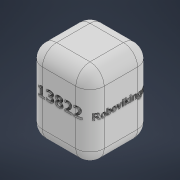
# Autodesk Inventor part: Robovikings Basic Capstone
Saved by Autodesk Inventor 2022 (Build 260153000, 153)
## iProperties
Created: 2022-01-25
Part Number: Robovikings Basic Capstone
Material: Generic
Document SubType Name: Modeling
Designer: izack
Density: 1 g/cm^3
Appearance: Default
Author: izack
Autodesk Inventor part; units mm, degrees
(part 1 of 2)
ref_plane "YZ Plane" through (0, 0, 0) normal (1, 0, 0) x (0, 1, 0)
ref_plane "XZ Plane" through (0, 0, 0) normal (0, 1, 0) x (-1, 0, 0)
ref_plane "XY Plane" through (0, 0, 0) normal (0, 0, 1) x (1, 0, 0)
sketch "Sketch1" plane through (0, 0, 0) normal (0, 1, 0) x (-1, 0, 0)
  line L0 (0, 0) -> (76.2, 0)
  line L1 (76.2, 0) -> (76.2, -76.2)
  line L2 (76.2, -76.2) -> (0, -76.2)
  line L3 (0, -76.2) -> (0, 0)
  dimension "d0" = 76.2
  dimension "d1" = 76.2
  constraints: 8 end point, 2 parallel, 1 horizontal, 1 perpendicular
  measures "d0" distance of L1.end L2.end
  measures "d1" distance of L0.end L1.end
extrude "Extrusion1" add sketch "Sketch1" along normal blind 101.6
shell "Shell1" thickness 12.7 removed faces 1 at (-25.4, 0, -25.4)
fillet "Fillet1" radius 17.4625 20 edges at (-38.1, 88.9, -63.5) (-63.5, 88.9, -38.1) (-63.5, 44.45, -63.5) (-63.5, 44.45, -12.7) (-12.7, 88.9, -38.1) (-38.1, 88.9, -12.7) (-12.7, 44.45, -63.5) (-12.7, 44.45, -12.7) (-38.1, 0, -76.2) (-76.2, 0, -38.1) (-38.1, 0, 0) (0, 0, -38.1) (-76.2, 50.8, -76.2) (-38.1, 101.6, -76.2) (-76.2, 101.6, -38.1) (0, 50.8, -76.2) (-76.2, 50.8, 0) (0, 50.8, 0) (-38.1, 101.6, 0) (0, 101.6, -38.1)
sketch "Sketch2" plane through (-76.2, 17.4625, -17.4625) normal (-1, 0, 0) x (0, 0, 1)
  line L0 (-41.275, 66.675) -> (-41.275, 0) projected
  line L1 (0, 0) -> (0, 66.675) projected
  line L2 (-41.275, 0) -> (-41.275, 66.675) projected
  line L3 (-41.275, 33.3375) -> (0, 33.3375)
  line L4 (-45.0845, 33.3375) -> (-47.4125, 33.3375)
  line L5 (-47.4125, 33.3375) -> (-49.5305, 36.1348)
  line L6 (-49.5305, 36.1348) -> (-50.2221, 36.1348)
  line L7 (-50.2221, 36.1348) -> (-50.2221, 33.3375)
  line L8 (-50.2221, 33.3375) -> (-52.124, 33.3375)
  line L9 (-52.124, 33.3375) -> (-52.124, 40.9575)
  line L10 (-52.124, 40.9575) -> (-49.0612, 40.9575)
  spline S0 degree 2 poles (-49.0612, 40.9575) (-48.4252, 40.9575) (-47.4866, 40.7969) (-47.0852, 40.5499) knots 0 0 0 1 2 2 2
  spline S1 degree 2 poles (-47.0852, 40.5499) (-46.6776, 40.2906) (-46.196, 39.4817) (-46.196, 38.8642) knots 0 0 0 1 2 2 2
  spline S2 degree 2 poles (-46.196, 38.8642) (-46.196, 37.9935) (-46.9864, 36.9005) (-47.6471, 36.5794) knots 0 0 0 1 2 2 2
  line L11 (-47.6471, 36.5794) -> (-45.0845, 33.3375)
  spline S3 degree 2 poles (-48.1597, 38.6233) (-48.1597, 38.9136) (-48.382, 39.3273) (-48.6351, 39.4384) knots 0 0 0 1 2 2 2
  spline S4 degree 2 poles (-48.6351, 39.4384) (-48.8142, 39.5125) (-49.2526, 39.5558) (-49.5799, 39.5558) knots 0 0 0 1 2 2 2
  line L12 (-49.5799, 39.5558) -> (-50.2221, 39.5558)
  line L13 (-50.2221, 39.5558) -> (-50.2221, 37.5057)
  line L14 (-50.2221, 37.5057) -> (-49.6725, 37.5057)
  spline S5 degree 2 poles (-49.6725, 37.5057) (-49.2773, 37.5057) (-48.7154, 37.6045) (-48.524, 37.7588) knots 0 0 0 1 2 2 2
  spline S6 degree 2 poles (-48.524, 37.7588) (-48.3387, 37.907) (-48.1597, 38.3022) (-48.1597, 38.6233) knots 0 0 0 1 2 2 2
  spline S7 degree 2 poles (-39.107, 36.2089) (-39.107, 34.7886) (-40.657, 33.1584) (-42.0711, 33.1584) knots 0 0 0 1 2 2 2
  spline S8 degree 2 poles (-42.0711, 33.1584) (-43.479, 33.1584) (-45.0413, 34.7886) (-45.0413, 36.2089) knots 0 0 0 1 2 2 2
  spline S9 degree 2 poles (-45.0413, 36.2089) (-45.0413, 37.6415) (-43.479, 39.2655) (-42.0711, 39.2655) knots 0 0 0 1 2 2 2
  spline S10 degree 2 poles (-42.0711, 39.2655) (-40.6632, 39.2655) (-39.107, 37.6353) (-39.107, 36.2089) knots 0 0 0 1 2 2 2
  spline S11 degree 2 poles (-40.941, 36.1965) (-40.941, 36.7091) (-41.1078, 37.3945) (-41.256, 37.5983) knots 0 0 0 1 2 2 2
  spline S12 degree 2 poles (-41.256, 37.5983) (-41.4165, 37.8144) (-41.8179, 37.9811) (-42.0711, 37.9811) knots 0 0 0 1 2 2 2
  spline S13 degree 2 poles (-42.0711, 37.9811) (-42.3181, 37.9811) (-42.7071, 37.8329) (-42.8676, 37.623) knots 0 0 0 1 2 2 2
  spline S14 degree 2 poles (-42.8676, 37.623) (-43.022, 37.4254) (-43.2073, 36.7276) (-43.2073, 36.1965) knots 0 0 0 1 2 2 2
  spline S15 degree 2 poles (-43.2073, 36.1965) (-43.2073, 35.6717) (-43.0344, 35.0233) (-42.8923, 34.8257) knots 0 0 0 1 2 2 2
  spline S16 degree 2 poles (-42.8923, 34.8257) (-42.7503, 34.6281) (-42.3181, 34.4428) (-42.0587, 34.4428) knots 0 0 0 1 2 2 2
  spline S17 degree 2 poles (-42.0587, 34.4428) (-41.8426, 34.4428) (-41.398, 34.6281) (-41.2621, 34.8133) knots 0 0 0 1 2 2 2
  spline S18 degree 2 poles (-41.2621, 34.8133) (-41.1078, 35.0295) (-40.941, 35.6531) (-40.941, 36.1965) knots 0 0 0 1 2 2 2
  spline S19 degree 2 poles (-32.5245, 36.2892) (-32.5245, 34.9183) (-33.9138, 33.2263) (-34.9451, 33.2263) knots 0 0 0 1 2 2 2
  spline S20 degree 2 poles (-34.9451, 33.2263) (-35.3711, 33.2263) (-36.0072, 33.4178) (-36.3653, 33.6216) knots 0 0 0 1 2 2 2
  line L15 (-36.3653, 33.6216) -> (-36.4394, 33.3375)
  line L16 (-36.4394, 33.3375) -> (-38.1561, 33.3375)
  line L17 (-38.1561, 33.3375) -> (-38.1561, 41.2971)
  line L18 (-38.1561, 41.2971) -> (-36.3653, 41.2971)
  line L19 (-36.3653, 41.2971) -> (-36.3653, 38.4813)
  spline S21 degree 2 poles (-36.3653, 38.4813) (-35.9701, 38.8209) (-35.155, 39.2408) (-34.6178, 39.2408) knots 0 0 0 1 2 2 2
  spline S22 degree 2 poles (-34.6178, 39.2408) (-33.6113, 39.2408) (-32.5245, 37.6786) (-32.5245, 36.2892) knots 0 0 0 1 2 2 2
  spline S23 degree 2 poles (-34.3584, 36.2521) (-34.3584, 37.1104) (-34.8771, 37.8453) (-35.4205, 37.8453) knots 0 0 0 1 2 2 2
  spline S24 degree 2 poles (-35.4205, 37.8453) (-35.6614, 37.8453) (-36.1369, 37.6909) (-36.3653, 37.5365) knots 0 0 0 1 2 2 2
  line L20 (-36.3653, 37.5365) -> (-36.3653, 34.659)
  spline S25 degree 2 poles (-36.3653, 34.659) (-36.1863, 34.5849) (-35.8219, 34.5355) (-35.6428, 34.5355) knots 0 0 0 1 2 2 2
  spline S26 degree 2 poles (-35.6428, 34.5355) (-34.9945, 34.5355) (-34.3584, 35.3938) (-34.3584, 36.2521) knots 0 0 0 1 2 2 2
  spline S27 degree 2 poles (-26.0221, 36.2089) (-26.0221, 34.7886) (-27.5721, 33.1584) (-28.9862, 33.1584) knots 0 0 0 1 2 2 2
  spline S28 degree 2 poles (-28.9862, 33.1584) (-30.3941, 33.1584) (-31.9563, 34.7886) (-31.9563, 36.2089) knots 0 0 0 1 2 2 2
  spline S29 degree 2 poles (-31.9563, 36.2089) (-31.9563, 37.6415) (-30.3941, 39.2655) (-28.9862, 39.2655) knots 0 0 0 1 2 2 2
  spline S30 degree 2 poles (-28.9862, 39.2655) (-27.5782, 39.2655) (-26.0221, 37.6353) (-26.0221, 36.2089) knots 0 0 0 1 2 2 2
  spline S31 degree 2 poles (-27.8561, 36.1965) (-27.8561, 36.7091) (-28.0228, 37.3945) (-28.171, 37.5983) knots 0 0 0 1 2 2 2
  spline S32 degree 2 poles (-28.171, 37.5983) (-28.3316, 37.8144) (-28.733, 37.9811) (-28.9862, 37.9811) knots 0 0 0 1 2 2 2
  spline S33 degree 2 poles (-28.9862, 37.9811) (-29.2332, 37.9811) (-29.6222, 37.8329) (-29.7827, 37.623) knots 0 0 0 1 2 2 2
  spline S34 degree 2 poles (-29.7827, 37.623) (-29.9371, 37.4254) (-30.1224, 36.7276) (-30.1224, 36.1965) knots 0 0 0 1 2 2 2
  spline S35 degree 2 poles (-30.1224, 36.1965) (-30.1224, 35.6717) (-29.9495, 35.0233) (-29.8074, 34.8257) knots 0 0 0 1 2 2 2
  spline S36 degree 2 poles (-29.8074, 34.8257) (-29.6654, 34.6281) (-29.2332, 34.4428) (-28.9738, 34.4428) knots 0 0 0 1 2 2 2
  spline S37 degree 2 poles (-28.9738, 34.4428) (-28.7577, 34.4428) (-28.3131, 34.6281) (-28.1772, 34.8133) knots 0 0 0 1 2 2 2
  spline S38 degree 2 poles (-28.1772, 34.8133) (-28.0228, 35.0295) (-27.8561, 35.6531) (-27.8561, 36.1965) knots 0 0 0 1 2 2 2
  line L21 (-19.6927, 39.0865) -> (-21.7552, 33.3375)
  line L22 (-21.7552, 33.3375) -> (-23.7127, 33.3375)
  line L23 (-23.7127, 33.3375) -> (-25.7566, 39.0865)
  line L24 (-25.7566, 39.0865) -> (-23.8732, 39.0865)
  line L25 (-23.8732, 39.0865) -> (-22.7, 35.2888)
  line L26 (-22.7, 35.2888) -> (-21.5391, 39.0865)
  line L27 (-21.5391, 39.0865) -> (-19.6927, 39.0865)
  line L28 (-17.2165, 33.3375) -> (-19.0073, 33.3375)
  line L29 (-19.0073, 33.3375) -> (-19.0073, 39.0865)
  line L30 (-19.0073, 39.0865) -> (-17.2165, 39.0865)
  line L31 (-17.2165, 39.0865) -> (-17.2165, 33.3375)
  line L32 (-17.161, 39.9077) -> (-19.0567, 39.9077)
  line L33 (-19.0567, 39.9077) -> (-19.0567, 41.3033)
  line L34 (-19.0567, 41.3033) -> (-17.161, 41.3033)
  line L35 (-17.161, 41.3033) -> (-17.161, 39.9077)
  line L36 (-10.0905, 33.3375) -> (-12.2209, 33.3375)
  line L37 (-12.2209, 33.3375) -> (-13.777, 35.8322)
  line L38 (-13.777, 35.8322) -> (-14.0549, 35.4617)
  line L39 (-14.0549, 35.4617) -> (-14.0549, 33.3375)
  line L40 (-14.0549, 33.3375) -> (-15.8457, 33.3375)
  line L41 (-15.8457, 33.3375) -> (-15.8457, 41.2971)
  line L42 (-15.8457, 41.2971) -> (-14.0549, 41.2971)
  line L43 (-14.0549, 41.2971) -> (-14.0549, 36.8387)
  line L44 (-14.0549, 36.8387) -> (-12.3568, 39.0865)
  line L45 (-12.3568, 39.0865) -> (-10.2387, 39.0865)
  line L46 (-10.2387, 39.0865) -> (-12.2518, 36.6103)
  line L47 (-12.2518, 36.6103) -> (-10.0905, 33.3375)
  line L48 (-7.7378, 33.3375) -> (-9.5286, 33.3375)
  line L49 (-9.5286, 33.3375) -> (-9.5286, 39.0865)
  line L50 (-9.5286, 39.0865) -> (-7.7378, 39.0865)
  line L51 (-7.7378, 39.0865) -> (-7.7378, 33.3375)
  line L52 (-7.6823, 39.9077) -> (-9.578, 39.9077)
  line L53 (-9.578, 39.9077) -> (-9.578, 41.3033)
  line L54 (-9.578, 41.3033) -> (-7.6823, 41.3033)
  line L55 (-7.6823, 41.3033) -> (-7.6823, 39.9077)
  line L56 (-0.9885, 33.3375) -> (-2.7916, 33.3375)
  line L57 (-2.7916, 33.3375) -> (-2.7916, 36.1842)
  spline S39 degree 2 poles (-2.7916, 36.1842) (-2.7916, 36.5362) (-2.8472, 37.2278) (-2.9213, 37.3883) knots 0 0 0 1 2 2 2
  spline S40 degree 2 poles (-2.9213, 37.3883) (-3.0139, 37.5859) (-3.3597, 37.7527) (-3.6561, 37.7527) knots 0 0 0 1 2 2 2
  spline S41 degree 2 poles (-3.6561, 37.7527) (-3.8723, 37.7527) (-4.323, 37.5859) (-4.5762, 37.4069) knots 0 0 0 1 2 2 2
  line L58 (-4.5762, 37.4069) -> (-4.5762, 33.3375)
  line L59 (-4.5762, 33.3375) -> (-6.367, 33.3375)
  line L60 (-6.367, 33.3375) -> (-6.367, 39.0865)
  line L61 (-6.367, 39.0865) -> (-4.5762, 39.0865)
  line L62 (-4.5762, 39.0865) -> (-4.5762, 38.4504)
  spline S42 degree 2 poles (-4.5762, 38.4504) (-4.1378, 38.8209) (-3.3042, 39.2408) (-2.7978, 39.2408) knots 0 0 0 1 2 2 2
  spline S43 degree 2 poles (-2.7978, 39.2408) (-1.921, 39.2408) (-0.9885, 38.1293) (-0.9885, 37.0796) knots 0 0 0 1 2 2 2
  line L63 (-0.9885, 37.0796) -> (-0.9885, 33.3375)
  spline S44 degree 2 poles (5.5632, 33.9982) (5.5632, 33.2016) (5.1001, 32.084) (4.7049, 31.7752) knots 0 0 0 1 2 2 2
  spline S45 degree 2 poles (4.7049, 31.7752) (4.3035, 31.4603) (3.192, 31.1762) (2.5127, 31.1762) knots 0 0 0 1 2 2 2
  spline S46 degree 2 poles (2.5127, 31.1762) (1.9384, 31.1762) (0.9072, 31.3244) (0.5305, 31.4232) knots 0 0 0 1 2 2 2
  line L64 (0.5305, 31.4232) -> (0.5305, 32.862)
  line L65 (0.5305, 32.862) -> (0.7405, 32.862)
  spline S47 degree 2 poles (0.7405, 32.862) (0.8702, 32.8126) (1.2345, 32.6891) (1.4197, 32.6397) knots 0 0 0 1 2 2 2
  spline S48 degree 2 poles (1.4197, 32.6397) (1.642, 32.5841) (2.0619, 32.51) (2.2781, 32.51) knots 0 0 0 1 2 2 2
  spline S49 degree 2 poles (2.2781, 32.51) (2.735, 32.51) (3.3402, 32.6953) (3.4946, 32.8682) knots 0 0 0 1 2 2 2
  spline S50 degree 2 poles (3.4946, 32.8682) (3.6489, 33.0473) (3.7724, 33.5289) (3.7724, 33.8994) knots 0 0 0 1 2 2 2
  line L66 (3.7724, 33.8994) -> (3.7724, 34.0044)
  spline S51 degree 2 poles (3.7724, 34.0044) (3.4699, 33.7389) (2.6795, 33.4178) (2.2596, 33.4178) knots 0 0 0 1 2 2 2
  spline S52 degree 2 poles (2.2596, 33.4178) (1.1419, 33.4178) (-0.0684, 34.8689) (-0.0684, 36.3571) knots 0 0 0 1 2 2 2
  spline S53 degree 2 poles (-0.0684, 36.3571) (-0.0684, 37.0302) (0.3021, 38.1046) (0.6355, 38.4813) knots 0 0 0 1 2 2 2
  spline S54 degree 2 poles (0.6355, 38.4813) (0.9566, 38.8456) (1.852, 39.2408) (2.3398, 39.2408) knots 0 0 0 1 2 2 2
  spline S55 degree 2 poles (2.3398, 39.2408) (2.7783, 39.2408) (3.476, 39.0185) (3.7601, 38.8333) knots 0 0 0 1 2 2 2
  line L67 (3.7601, 38.8333) -> (3.828, 39.0865)
  line L68 (3.828, 39.0865) -> (5.5632, 39.0865)
  line L69 (5.5632, 39.0865) -> (5.5632, 33.9982)
  line L70 (3.7724, 35.1468) -> (3.7724, 37.7527)
  spline S56 degree 2 poles (3.7724, 37.7527) (3.6428, 37.8144) (3.2537, 37.8947) (3.0561, 37.8947) knots 0 0 0 1 2 2 2
  spline S57 degree 2 poles (3.0561, 37.8947) (2.4139, 37.8947) (1.7655, 37.061) (1.7655, 36.3139) knots 0 0 0 1 2 2 2
  spline S58 degree 2 poles (1.7655, 36.3139) (1.7655, 35.9434) (1.8643, 35.4247) (1.994, 35.2271) knots 0 0 0 1 2 2 2
  spline S59 degree 2 poles (1.994, 35.2271) (2.1237, 35.0295) (2.5374, 34.8319) (2.8585, 34.8319) knots 0 0 0 1 2 2 2
  spline S60 degree 2 poles (2.8585, 34.8319) (3.0994, 34.8319) (3.5625, 34.9986) (3.7724, 35.1468) knots 0 0 0 1 2 2 2
  spline S61 degree 2 poles (8.6816, 33.1831) (8.0517, 33.1831) (6.9217, 33.461) (6.5512, 33.6463) knots 0 0 0 1 2 2 2
  line L71 (6.5512, 33.6463) -> (6.5512, 35.1591)
  line L72 (6.5512, 35.1591) -> (6.6994, 35.1591)
  spline S62 degree 2 poles (6.6994, 35.1591) (6.8291, 35.0603) (7.1564, 34.8257) (7.4466, 34.696) knots 0 0 0 1 2 2 2
  spline S63 degree 2 poles (7.4466, 34.696) (7.6998, 34.5787) (8.3234, 34.412) (8.6939, 34.412) knots 0 0 0 1 2 2 2
  spline S64 degree 2 poles (8.6939, 34.412) (9.0706, 34.412) (9.6511, 34.6466) (9.6511, 34.8998) knots 0 0 0 1 2 2 2
  spline S65 degree 2 poles (9.6511, 34.8998) (9.6511, 35.0974) (9.3855, 35.3073) (9.0027, 35.3938) knots 0 0 0 1 2 2 2
  spline S66 degree 2 poles (9.0027, 35.3938) (8.7989, 35.4494) (8.1752, 35.5667) (7.9344, 35.6408) knots 0 0 0 1 2 2 2
  spline S67 degree 2 poles (7.9344, 35.6408) (7.2552, 35.8507) (6.5759, 36.672) (6.5759, 37.3451) knots 0 0 0 1 2 2 2
  spline S68 degree 2 poles (6.5759, 37.3451) (6.5759, 37.728) (6.9279, 38.4072) (7.2737, 38.6727) knots 0 0 0 1 2 2 2
  spline S69 degree 2 poles (7.2737, 38.6727) (7.6133, 38.9321) (8.6198, 39.2408) (9.2559, 39.2408) knots 0 0 0 1 2 2 2
  spline S70 degree 2 poles (9.2559, 39.2408) (9.861, 39.2408) (10.8737, 39) (11.2195, 38.8333) knots 0 0 0 1 2 2 2
  line L73 (11.2195, 38.8333) -> (11.2195, 37.376)
  line L74 (11.2195, 37.376) -> (11.0775, 37.376)
  spline S71 degree 2 poles (11.0775, 37.376) (10.9849, 37.4501) (10.5835, 37.6909) (10.3983, 37.7774) knots 0 0 0 1 2 2 2
  spline S72 degree 2 poles (10.3983, 37.7774) (10.1698, 37.8762) (9.614, 38.012) (9.3238, 38.012) knots 0 0 0 1 2 2 2
  spline S73 degree 2 poles (9.3238, 38.012) (8.9348, 38.012) (8.3975, 37.7465) (8.3975, 37.5304) knots 0 0 0 1 2 2 2
  spline S74 degree 2 poles (8.3975, 37.5304) (8.3975, 37.3328) (8.6631, 37.1104) (9.1077, 36.9993) knots 0 0 0 1 2 2 2
  spline S75 degree 2 poles (9.1077, 36.9993) (9.3361, 36.9437) (9.9351, 36.8387) (10.213, 36.7461) knots 0 0 0 1 2 2 2
  spline S76 degree 2 poles (10.213, 36.7461) (10.8305, 36.5485) (11.4727, 35.7766) (11.4727, 35.1344) knots 0 0 0 1 2 2 2
  spline S77 degree 2 poles (11.4727, 35.1344) (11.4727, 34.7331) (11.096, 33.9982) (10.7441, 33.7512) knots 0 0 0 1 2 2 2
  spline S78 degree 2 poles (10.7441, 33.7512) (10.3797, 33.4795) (9.3794, 33.1831) (8.6816, 33.1831) knots 0 0 0 1 2 2 2
  point P0 (17.4625, -17.4625)
  constraints: 2 end point, 2 midpoint, 1 horizontal
extrude "Extrusion2" cut sketch "Sketch2" against normal blind 5.08 contours S10 S7 L3 L0 S17 S18 S11 S12 | L0 S12 S13 S14 S15 S16 S17 S7 S8 S9 S10 | S7 L0 L3 | S52 S53 L1 | L1 S53 S54 S55 L67 L68 L69 S44 S45 S46 L64 L65 S47 S48 S49 S50 L66 S51 S52 | L17 L18 L19 S21 S22 S19 L3 S20 L15 | L3 S19 S20 | L23 L24 L25 L26 L27 L21 L3 | L29 L30 L31 L3 | L41 L42 L43 L44 L45 L46 L47 L3 L37 L38 L39 | L49 L50 L51 L3 | L60 L61 L62 S42 S43 L63 L3 L57 S39 S40 S41 L58 | S28 S29 S30 S27 L3 | L3 S27 S28 | L4 L5 L6 L7 L8 L9 L10 S0 S1 S2 L11 | L32 L33 L34 L35 | L52 L53 L54 L55 | S61 L71 L72 S62 S63 S64 S65 S66 S67 S68 S69 S70 L73 L74 S71 S72 S73 S74 S75 S76 S77 S78
sketch "Sketch3" plane through (-58.7375, 17.4625, 0) normal (0, 0, 1) x (1, 0, 0)
  line L0 (0, 66.675) -> (0, 0) projected
  line L1 (0, 33.3375) -> (41.275, 33.3375)
  line L2 (41.275, 0) -> (41.275, 66.675) projected
  line L3 (2.8791, 33.3375) -> (-5.5086, 33.3375)
  line L4 (-5.5086, 33.3375) -> (-5.5086, 35.5502)
  line L5 (-5.5086, 35.5502) -> (-2.8328, 35.5502)
  line L6 (-2.8328, 35.5502) -> (-2.8328, 42.2707)
  line L7 (-2.8328, 42.2707) -> (-5.5086, 42.2707)
  line L8 (-5.5086, 42.2707) -> (-5.5086, 44.3394)
  spline S0 degree 2 poles (-5.5086, 44.3394) (-4.922, 44.3394) (-3.7591, 44.4937) (-3.4091, 44.6584) knots 0 0 0 1 2 2 2
  spline S1 degree 2 poles (-3.4091, 44.6584) (-3.0078, 44.8642) (-2.5549, 45.5538) (-2.5138, 46.0684) knots 0 0 0 1 2 2 2
  line L9 (-2.5138, 46.0684) -> (0.265, 46.0684)
  line L10 (0.265, 46.0684) -> (0.265, 35.5502)
  line L11 (0.265, 35.5502) -> (2.8791, 35.5502)
  line L12 (2.8791, 35.5502) -> (2.8791, 33.3375)
  spline S2 degree 2 poles (14.2515, 37.1866) (14.2515, 36.2501) (13.5619, 34.7166) (12.893, 34.1814) knots 0 0 0 1 2 2 2
  spline S3 degree 2 poles (12.893, 34.1814) (12.224, 33.6463) (10.4024, 33.0699) (9.0953, 33.0699) knots 0 0 0 1 2 2 2
  spline S4 degree 2 poles (9.0953, 33.0699) (7.6133, 33.0699) (5.4932, 33.5639) (4.8243, 33.8727) knots 0 0 0 1 2 2 2
  line L13 (4.8243, 33.8727) -> (4.8243, 36.6309)
  line L14 (4.8243, 36.6309) -> (5.133, 36.6309)
  spline S5 degree 2 poles (5.133, 36.6309) (5.8328, 36.1883) (7.7162, 35.5296) (8.4984, 35.5296) knots 0 0 0 1 2 2 2
  spline S6 degree 2 poles (8.4984, 35.5296) (8.9615, 35.5296) (10.0422, 35.6943) (10.4127, 35.9619) knots 0 0 0 1 2 2 2
  spline S7 degree 2 poles (10.4127, 35.9619) (10.7008, 36.178) (11.0508, 36.8058) (11.0508, 37.3719) knots 0 0 0 1 2 2 2
  spline S8 degree 2 poles (11.0508, 37.3719) (11.0508, 37.9379) (10.5567, 38.5451) (10.1451, 38.6892) knots 0 0 0 1 2 2 2
  spline S9 degree 2 poles (10.1451, 38.6892) (9.7334, 38.8333) (8.591, 38.8642) (8.1485, 38.8642) knots 0 0 0 1 2 2 2
  line L15 (8.1485, 38.8642) -> (7.603, 38.8642)
  line L16 (7.603, 38.8642) -> (7.603, 41.0975)
  line L17 (7.603, 41.0975) -> (8.1073, 41.0975)
  spline S10 degree 2 poles (8.1073, 41.0975) (8.6837, 41.0975) (9.6614, 41.2004) (10.001, 41.3548) knots 0 0 0 1 2 2 2
  spline S11 degree 2 poles (10.001, 41.3548) (10.3406, 41.5194) (10.7214, 42.0958) (10.7214, 42.5898) knots 0 0 0 1 2 2 2
  spline S12 degree 2 poles (10.7214, 42.5898) (10.7214, 42.9809) (10.3612, 43.4646) (10.1039, 43.5984) knots 0 0 0 1 2 2 2
  spline S13 degree 2 poles (10.1039, 43.5984) (9.7952, 43.7527) (8.9718, 43.8557) (8.6837, 43.8557) knots 0 0 0 1 2 2 2
  spline S14 degree 2 poles (8.6837, 43.8557) (8.2205, 43.8557) (7.2428, 43.6395) (6.79, 43.4646) knots 0 0 0 1 2 2 2
  spline S15 degree 2 poles (6.79, 43.4646) (6.4298, 43.3308) (5.6476, 42.8985) (5.4623, 42.7853) knots 0 0 0 1 2 2 2
  line L18 (5.4623, 42.7853) -> (5.1948, 42.7853)
  line L19 (5.1948, 42.7853) -> (5.1948, 45.5023)
  spline S16 degree 2 poles (5.1948, 45.5023) (5.8534, 45.7802) (8.0764, 46.3051) (9.2394, 46.3051) knots 0 0 0 1 2 2 2
  spline S17 degree 2 poles (9.2394, 46.3051) (10.3715, 46.3051) (12.0388, 45.914) (12.6254, 45.5332) knots 0 0 0 1 2 2 2
  spline S18 degree 2 poles (12.6254, 45.5332) (13.2738, 45.1318) (13.9221, 43.8968) (13.9221, 43.1249) knots 0 0 0 1 2 2 2
  spline S19 degree 2 poles (13.9221, 43.1249) (13.9221, 42.034) (12.6666, 40.4079) (11.6374, 40.1712) knots 0 0 0 1 2 2 2
  line L20 (11.6374, 40.1712) -> (11.6374, 40.0477)
  spline S20 degree 2 poles (11.6374, 40.0477) (12.0902, 39.986) (12.9547, 39.6566) (13.3664, 39.2861) knots 0 0 0 1 2 2 2
  spline S21 degree 2 poles (13.3664, 39.2861) (13.7472, 38.9568) (14.2515, 37.907) (14.2515, 37.1866) knots 0 0 0 1 2 2 2
  spline S22 degree 2 poles (25.665, 36.8676) (25.665, 36.0545) (24.9858, 34.6446) (24.3374, 34.13) knots 0 0 0 1 2 2 2
  spline S23 degree 2 poles (24.3374, 34.13) (23.689, 33.6154) (21.8262, 33.039) (20.6221, 33.039) knots 0 0 0 1 2 2 2
  spline S24 degree 2 poles (20.6221, 33.039) (19.3356, 33.039) (17.411, 33.6257) (16.7935, 34.13) knots 0 0 0 1 2 2 2
  spline S25 degree 2 poles (16.7935, 34.13) (16.1863, 34.6343) (15.61, 36.0031) (15.61, 36.7646) knots 0 0 0 1 2 2 2
  spline S26 degree 2 poles (15.61, 36.7646) (15.61, 37.8556) (16.8141, 39.3067) (17.9565, 39.7904) knots 0 0 0 1 2 2 2
  line L21 (17.9565, 39.7904) -> (17.9565, 39.8419)
  spline S27 degree 2 poles (17.9565, 39.8419) (16.8347, 40.3873) (15.9496, 41.9414) (15.9496, 42.8985) knots 0 0 0 1 2 2 2
  spline S28 degree 2 poles (15.9496, 42.8985) (15.9496, 43.5984) (16.5671, 44.8231) (17.1743, 45.3068) knots 0 0 0 1 2 2 2
  spline S29 degree 2 poles (17.1743, 45.3068) (17.761, 45.7699) (19.5414, 46.3257) (20.6529, 46.3257) knots 0 0 0 1 2 2 2
  spline S30 degree 2 poles (20.6529, 46.3257) (21.8262, 46.3257) (23.5758, 45.8214) (24.1418, 45.4097) knots 0 0 0 1 2 2 2
  spline S31 degree 2 poles (24.1418, 45.4097) (24.7182, 44.998) (25.3357, 43.8042) (25.3357, 43.1146) knots 0 0 0 1 2 2 2
  spline S32 degree 2 poles (25.3357, 43.1146) (25.3357, 42.209) (24.2859, 40.7578) (23.2053, 40.2535) knots 0 0 0 1 2 2 2
  line L22 (23.2053, 40.2535) -> (23.2053, 40.2124)
  spline S33 degree 2 poles (23.2053, 40.2124) (24.4712, 39.6978) (25.665, 38.0305) (25.665, 36.8676) knots 0 0 0 1 2 2 2
  spline S34 degree 2 poles (22.5157, 36.7338) (22.5157, 37.3616) (21.9806, 38.0202) (21.1161, 38.4422) knots 0 0 0 1 2 2 2
  spline S35 degree 2 poles (21.1161, 38.4422) (20.8691, 38.5554) (19.9325, 38.9156) (19.5723, 39.07) knots 0 0 0 1 2 2 2
  spline S36 degree 2 poles (19.5723, 39.07) (19.243, 38.7407) (18.7181, 37.7527) (18.7181, 37.166) knots 0 0 0 1 2 2 2
  spline S37 degree 2 poles (18.7181, 37.166) (18.7181, 36.2809) (19.8502, 35.2209) (20.7661, 35.2209) knots 0 0 0 1 2 2 2
  spline S38 degree 2 poles (20.7661, 35.2209) (21.0234, 35.2209) (21.6615, 35.3856) (21.9085, 35.5502) knots 0 0 0 1 2 2 2
  spline S39 degree 2 poles (21.9085, 35.5502) (22.1864, 35.7458) (22.5157, 36.2809) (22.5157, 36.7338) knots 0 0 0 1 2 2 2
  spline S40 degree 2 poles (22.2379, 42.7441) (22.2379, 43.3925) (21.3837, 44.1644) (20.6529, 44.1644) knots 0 0 0 1 2 2 2
  spline S41 degree 2 poles (20.6529, 44.1644) (19.9531, 44.1644) (19.0989, 43.4646) (19.0989, 42.95) knots 0 0 0 1 2 2 2
  spline S42 degree 2 poles (19.0989, 42.95) (19.0989, 42.4457) (19.6135, 41.8179) (20.1589, 41.5606) knots 0 0 0 1 2 2 2
  spline S43 degree 2 poles (20.1589, 41.5606) (20.3956, 41.4371) (21.0543, 41.1798) (21.5998, 40.974) knots 0 0 0 1 2 2 2
  spline S44 degree 2 poles (21.5998, 40.974) (21.9291, 41.4062) (22.2379, 42.2193) (22.2379, 42.7441) knots 0 0 0 1 2 2 2
  line L23 (36.8213, 33.3375) -> (27.4866, 33.3375)
  line L24 (27.4866, 33.3375) -> (27.4866, 35.4061)
  spline S45 degree 2 poles (27.4866, 35.4061) (28.6702, 36.353) (30.5639, 38.0202) (31.274, 38.7715) knots 0 0 0 1 2 2 2
  spline S46 degree 2 poles (31.274, 38.7715) (32.2106, 39.7493) (33.0442, 41.2416) (33.0442, 42.0237) knots 0 0 0 1 2 2 2
  spline S47 degree 2 poles (33.0442, 42.0237) (33.0442, 42.9088) (31.9841, 43.8557) (31.0373, 43.8557) knots 0 0 0 1 2 2 2
  spline S48 degree 2 poles (31.0373, 43.8557) (30.5536, 43.8557) (29.6891, 43.6189) (29.2465, 43.4337) knots 0 0 0 1 2 2 2
  spline S49 degree 2 poles (29.2465, 43.4337) (28.8143, 43.2381) (28.1968, 42.8265) (28.0424, 42.7236) knots 0 0 0 1 2 2 2
  line L25 (28.0424, 42.7236) -> (27.7954, 42.7236)
  line L26 (27.7954, 42.7236) -> (27.7954, 45.492)
  spline S50 degree 2 poles (27.7954, 45.492) (28.3306, 45.7493) (30.6153, 46.2845) (31.6754, 46.2845) knots 0 0 0 1 2 2 2
  spline S51 degree 2 poles (31.6754, 46.2845) (33.9396, 46.2845) (36.2655, 44.2673) (36.2655, 42.4457) knots 0 0 0 1 2 2 2
  spline S52 degree 2 poles (36.2655, 42.4457) (36.2655, 41.3239) (35.2054, 39.1626) (33.9807, 37.9276) knots 0 0 0 1 2 2 2
  spline S53 degree 2 poles (33.9807, 37.9276) (33.2089, 37.166) (31.7577, 35.9825) (31.4387, 35.7355) knots 0 0 0 1 2 2 2
  line L27 (31.4387, 35.7355) -> (36.8213, 35.7355)
  line L28 (36.8213, 35.7355) -> (36.8213, 33.3375)
  line L29 (47.9466, 33.3375) -> (38.612, 33.3375)
  line L30 (38.612, 33.3375) -> (38.612, 35.4061)
  spline S54 degree 2 poles (38.612, 35.4061) (39.7956, 36.353) (41.6892, 38.0202) (42.3994, 38.7715) knots 0 0 0 1 2 2 2
  spline S55 degree 2 poles (42.3994, 38.7715) (43.3359, 39.7493) (44.1695, 41.2416) (44.1695, 42.0237) knots 0 0 0 1 2 2 2
  spline S56 degree 2 poles (44.1695, 42.0237) (44.1695, 42.9088) (43.1095, 43.8557) (42.1627, 43.8557) knots 0 0 0 1 2 2 2
  spline S57 degree 2 poles (42.1627, 43.8557) (41.6789, 43.8557) (40.8144, 43.6189) (40.3719, 43.4337) knots 0 0 0 1 2 2 2
  spline S58 degree 2 poles (40.3719, 43.4337) (39.9396, 43.2381) (39.3221, 42.8265) (39.1678, 42.7236) knots 0 0 0 1 2 2 2
  line L31 (39.1678, 42.7236) -> (38.9208, 42.7236)
  line L32 (38.9208, 42.7236) -> (38.9208, 45.492)
  spline S59 degree 2 poles (38.9208, 45.492) (39.4559, 45.7493) (41.7407, 46.2845) (42.8007, 46.2845) knots 0 0 0 1 2 2 2
  spline S60 degree 2 poles (42.8007, 46.2845) (45.0649, 46.2845) (47.3909, 44.2673) (47.3909, 42.4457) knots 0 0 0 1 2 2 2
  spline S61 degree 2 poles (47.3909, 42.4457) (47.3909, 41.3239) (46.3308, 39.1626) (45.1061, 37.9276) knots 0 0 0 1 2 2 2
  spline S62 degree 2 poles (45.1061, 37.9276) (44.3342, 37.166) (42.8831, 35.9825) (42.564, 35.7355) knots 0 0 0 1 2 2 2
  line L33 (42.564, 35.7355) -> (47.9466, 35.7355)
  line L34 (47.9466, 35.7355) -> (47.9466, 33.3375)
  point P0 (58.7375, -17.4625)
  constraints: 2 end point, 2 midpoint, 1 horizontal
extrude "Extrusion3" cut sketch "Sketch3" against normal blind 5.08 contours L9 L10 L11 L12 L1 L0 | L0 L3 L4 L5 L6 L7 L8 S0 S1 L9 | L24 S45 S46 S47 S48 S49 L25 L26 S50 S51 S52 S53 L27 L28 L1 | L30 S54 L2 L1 | L2 S54 S55 S56 S57 S59 S60 S61 S62 L33 L34 L29 | S57 S58 L31 L32 S59 L2 | S4 L13 L14 S5 S6 S7 S8 S9 L15 L16 L17 S10 S11 S12 S13 S14 S15 L18 L19 S16 S17 S18 S19 L20 S20 S21 S2 S3 L1 | L1 S3 S4 | S24 S25 S26 L21 S27 S28 S29 S30 S31 S32 L22 S33 S22 S23 L1 | L1 S23 S24
sketch "Sketch4" plane through (0, 17.4625, -58.7375) normal (1, 0, 0) x (0, 0, -1)
  line L0 (-41.275, 66.675) -> (-41.275, 0)
  line L1 (0, 0) -> (0, 66.675)
  line L2 (-41.275, 0) -> (-41.275, 66.675)
  line L3 (-41.275, 33.3375) -> (0, 33.3375)
  line L4 (-45.0845, 33.3375) -> (-47.4125, 33.3375)
  line L5 (-47.4125, 33.3375) -> (-49.5305, 36.1348)
  line L6 (-49.5305, 36.1348) -> (-50.2221, 36.1348)
  line L7 (-50.2221, 36.1348) -> (-50.2221, 33.3375)
  line L8 (-50.2221, 33.3375) -> (-52.124, 33.3375)
  line L9 (-52.124, 33.3375) -> (-52.124, 40.9575)
  line L10 (-52.124, 40.9575) -> (-49.0612, 40.9575)
  spline S0 degree 2 poles (-49.0612, 40.9575) (-48.4252, 40.9575) (-47.4866, 40.7969) (-47.0852, 40.5499) knots 0 0 0 1 2 2 2
  spline S1 degree 2 poles (-47.0852, 40.5499) (-46.6776, 40.2906) (-46.196, 39.4817) (-46.196, 38.8642) knots 0 0 0 1 2 2 2
  spline S2 degree 2 poles (-46.196, 38.8642) (-46.196, 37.9935) (-46.9864, 36.9005) (-47.6471, 36.5794) knots 0 0 0 1 2 2 2
  line L11 (-47.6471, 36.5794) -> (-45.0845, 33.3375)
  spline S3 degree 2 poles (-48.1597, 38.6233) (-48.1597, 38.9136) (-48.382, 39.3273) (-48.6351, 39.4384) knots 0 0 0 1 2 2 2
  spline S4 degree 2 poles (-48.6351, 39.4384) (-48.8142, 39.5125) (-49.2526, 39.5558) (-49.5799, 39.5558) knots 0 0 0 1 2 2 2
  line L12 (-49.5799, 39.5558) -> (-50.2221, 39.5558)
  line L13 (-50.2221, 39.5558) -> (-50.2221, 37.5057)
  line L14 (-50.2221, 37.5057) -> (-49.6725, 37.5057)
  spline S5 degree 2 poles (-49.6725, 37.5057) (-49.2773, 37.5057) (-48.7154, 37.6045) (-48.524, 37.7588) knots 0 0 0 1 2 2 2
  spline S6 degree 2 poles (-48.524, 37.7588) (-48.3387, 37.907) (-48.1597, 38.3022) (-48.1597, 38.6233) knots 0 0 0 1 2 2 2
  spline S7 degree 2 poles (-39.107, 36.2089) (-39.107, 34.7886) (-40.657, 33.1584) (-42.0711, 33.1584) knots 0 0 0 1 2 2 2
  spline S8 degree 2 poles (-42.0711, 33.1584) (-43.479, 33.1584) (-45.0413, 34.7886) (-45.0413, 36.2089) knots 0 0 0 1 2 2 2
  spline S9 degree 2 poles (-45.0413, 36.2089) (-45.0413, 37.6415) (-43.479, 39.2655) (-42.0711, 39.2655) knots 0 0 0 1 2 2 2
  spline S10 degree 2 poles (-42.0711, 39.2655) (-40.6632, 39.2655) (-39.107, 37.6353) (-39.107, 36.2089) knots 0 0 0 1 2 2 2
  spline S11 degree 2 poles (-40.941, 36.1965) (-40.941, 36.7091) (-41.1078, 37.3945) (-41.256, 37.5983) knots 0 0 0 1 2 2 2
  spline S12 degree 2 poles (-41.256, 37.5983) (-41.4165, 37.8144) (-41.8179, 37.9811) (-42.0711, 37.9811) knots 0 0 0 1 2 2 2
  spline S13 degree 2 poles (-42.0711, 37.9811) (-42.3181, 37.9811) (-42.7071, 37.8329) (-42.8676, 37.623) knots 0 0 0 1 2 2 2
  spline S14 degree 2 poles (-42.8676, 37.623) (-43.022, 37.4254) (-43.2073, 36.7276) (-43.2073, 36.1965) knots 0 0 0 1 2 2 2
  spline S15 degree 2 poles (-43.2073, 36.1965) (-43.2073, 35.6717) (-43.0344, 35.0233) (-42.8923, 34.8257) knots 0 0 0 1 2 2 2
  spline S16 degree 2 poles (-42.8923, 34.8257) (-42.7503, 34.6281) (-42.3181, 34.4428) (-42.0587, 34.4428) knots 0 0 0 1 2 2 2
  spline S17 degree 2 poles (-42.0587, 34.4428) (-41.8426, 34.4428) (-41.398, 34.6281) (-41.2621, 34.8133) knots 0 0 0 1 2 2 2
  spline S18 degree 2 poles (-41.2621, 34.8133) (-41.1078, 35.0295) (-40.941, 35.6531) (-40.941, 36.1965) knots 0 0 0 1 2 2 2
  spline S19 degree 2 poles (-32.5245, 36.2892) (-32.5245, 34.9183) (-33.9138, 33.2263) (-34.9451, 33.2263) knots 0 0 0 1 2 2 2
  spline S20 degree 2 poles (-34.9451, 33.2263) (-35.3711, 33.2263) (-36.0072, 33.4178) (-36.3653, 33.6216) knots 0 0 0 1 2 2 2
  line L15 (-36.3653, 33.6216) -> (-36.4394, 33.3375)
  line L16 (-36.4394, 33.3375) -> (-38.1561, 33.3375)
  line L17 (-38.1561, 33.3375) -> (-38.1561, 41.2971)
  line L18 (-38.1561, 41.2971) -> (-36.3653, 41.2971)
  line L19 (-36.3653, 41.2971) -> (-36.3653, 38.4813)
  spline S21 degree 2 poles (-36.3653, 38.4813) (-35.9701, 38.8209) (-35.155, 39.2408) (-34.6178, 39.2408) knots 0 0 0 1 2 2 2
  spline S22 degree 2 poles (-34.6178, 39.2408) (-33.6113, 39.2408) (-32.5245, 37.6786) (-32.5245, 36.2892) knots 0 0 0 1 2 2 2
  spline S23 degree 2 poles (-34.3584, 36.2521) (-34.3584, 37.1104) (-34.8771, 37.8453) (-35.4205, 37.8453) knots 0 0 0 1 2 2 2
  spline S24 degree 2 poles (-35.4205, 37.8453) (-35.6614, 37.8453) (-36.1369, 37.6909) (-36.3653, 37.5365) knots 0 0 0 1 2 2 2
  line L20 (-36.3653, 37.5365) -> (-36.3653, 34.659)
  spline S25 degree 2 poles (-36.3653, 34.659) (-36.1863, 34.5849) (-35.8219, 34.5355) (-35.6428, 34.5355) knots 0 0 0 1 2 2 2
  spline S26 degree 2 poles (-35.6428, 34.5355) (-34.9945, 34.5355) (-34.3584, 35.3938) (-34.3584, 36.2521) knots 0 0 0 1 2 2 2
  spline S27 degree 2 poles (-26.0221, 36.2089) (-26.0221, 34.7886) (-27.5721, 33.1584) (-28.9862, 33.1584) knots 0 0 0 1 2 2 2
  spline S28 degree 2 poles (-28.9862, 33.1584) (-30.3941, 33.1584) (-31.9563, 34.7886) (-31.9563, 36.2089) knots 0 0 0 1 2 2 2
  spline S29 degree 2 poles (-31.9563, 36.2089) (-31.9563, 37.6415) (-30.3941, 39.2655) (-28.9862, 39.2655) knots 0 0 0 1 2 2 2
  spline S30 degree 2 poles (-28.9862, 39.2655) (-27.5782, 39.2655) (-26.0221, 37.6353) (-26.0221, 36.2089) knots 0 0 0 1 2 2 2
  spline S31 degree 2 poles (-27.8561, 36.1965) (-27.8561, 36.7091) (-28.0228, 37.3945) (-28.171, 37.5983) knots 0 0 0 1 2 2 2
  spline S32 degree 2 poles (-28.171, 37.5983) (-28.3316, 37.8144) (-28.733, 37.9811) (-28.9862, 37.9811) knots 0 0 0 1 2 2 2
  spline S33 degree 2 poles (-28.9862, 37.9811) (-29.2332, 37.9811) (-29.6222, 37.8329) (-29.7827, 37.623) knots 0 0 0 1 2 2 2
  spline S34 degree 2 poles (-29.7827, 37.623) (-29.9371, 37.4254) (-30.1224, 36.7276) (-30.1224, 36.1965) knots 0 0 0 1 2 2 2
  spline S35 degree 2 poles (-30.1224, 36.1965) (-30.1224, 35.6717) (-29.9495, 35.0233) (-29.8074, 34.8257) knots 0 0 0 1 2 2 2
  spline S36 degree 2 poles (-29.8074, 34.8257) (-29.6654, 34.6281) (-29.2332, 34.4428) (-28.9738, 34.4428) knots 0 0 0 1 2 2 2
  spline S37 degree 2 poles (-28.9738, 34.4428) (-28.7577, 34.4428) (-28.3131, 34.6281) (-28.1772, 34.8133) knots 0 0 0 1 2 2 2
  spline S38 degree 2 poles (-28.1772, 34.8133) (-28.0228, 35.0295) (-27.8561, 35.6531) (-27.8561, 36.1965) knots 0 0 0 1 2 2 2
  line L21 (-19.6927, 39.0865) -> (-21.7552, 33.3375)
  line L22 (-21.7552, 33.3375) -> (-23.7127, 33.3375)
  line L23 (-23.7127, 33.3375) -> (-25.7566, 39.0865)
  line L24 (-25.7566, 39.0865) -> (-23.8732, 39.0865)
  line L25 (-23.8732, 39.0865) -> (-22.7, 35.2888)
  line L26 (-22.7, 35.2888) -> (-21.5391, 39.0865)
  line L27 (-21.5391, 39.0865) -> (-19.6927, 39.0865)
  line L28 (-17.2165, 33.3375) -> (-19.0073, 33.3375)
  line L29 (-19.0073, 33.3375) -> (-19.0073, 39.0865)
  line L30 (-19.0073, 39.0865) -> (-17.2165, 39.0865)
  line L31 (-17.2165, 39.0865) -> (-17.2165, 33.3375)
  line L32 (-17.161, 39.9077) -> (-19.0567, 39.9077)
  line L33 (-19.0567, 39.9077) -> (-19.0567, 41.3033)
  line L34 (-19.0567, 41.3033) -> (-17.161, 41.3033)
  line L35 (-17.161, 41.3033) -> (-17.161, 39.9077)
  line L36 (-10.0905, 33.3375) -> (-12.2209, 33.3375)
  line L37 (-12.2209, 33.3375) -> (-13.777, 35.8322)
  line L38 (-13.777, 35.8322) -> (-14.0549, 35.4617)
  line L39 (-14.0549, 35.4617) -> (-14.0549, 33.3375)
  line L40 (-14.0549, 33.3375) -> (-15.8457, 33.3375)
  line L41 (-15.8457, 33.3375) -> (-15.8457, 41.2971)
  line L42 (-15.8457, 41.2971) -> (-14.0549, 41.2971)
  line L43 (-14.0549, 41.2971) -> (-14.0549, 36.8387)
  line L44 (-14.0549, 36.8387) -> (-12.3568, 39.0865)
  line L45 (-12.3568, 39.0865) -> (-10.2387, 39.0865)
  line L46 (-10.2387, 39.0865) -> (-12.2518, 36.6103)
  line L47 (-12.2518, 36.6103) -> (-10.0905, 33.3375)
  line L48 (-7.7378, 33.3375) -> (-9.5286, 33.3375)
  line L49 (-9.5286, 33.3375) -> (-9.5286, 39.0865)
  line L50 (-9.5286, 39.0865) -> (-7.7378, 39.0865)
  line L51 (-7.7378, 39.0865) -> (-7.7378, 33.3375)
  line L52 (-7.6823, 39.9077) -> (-9.578, 39.9077)
  line L53 (-9.578, 39.9077) -> (-9.578, 41.3033)
  line L54 (-9.578, 41.3033) -> (-7.6823, 41.3033)
  line L55 (-7.6823, 41.3033) -> (-7.6823, 39.9077)
  line L56 (-0.9885, 33.3375) -> (-2.7916, 33.3375)
  line L57 (-2.7916, 33.3375) -> (-2.7916, 36.1842)
  spline S39 degree 2 poles (-2.7916, 36.1842) (-2.7916, 36.5362) (-2.8472, 37.2278) (-2.9213, 37.3883) knots 0 0 0 1 2 2 2
  spline S40 degree 2 poles (-2.9213, 37.3883) (-3.0139, 37.5859) (-3.3597, 37.7527) (-3.6561, 37.7527) knots 0 0 0 1 2 2 2
  spline S41 degree 2 poles (-3.6561, 37.7527) (-3.8723, 37.7527) (-4.323, 37.5859) (-4.5762, 37.4069) knots 0 0 0 1 2 2 2
  line L58 (-4.5762, 37.4069) -> (-4.5762, 33.3375)
  line L59 (-4.5762, 33.3375) -> (-6.367, 33.3375)
  line L60 (-6.367, 33.3375) -> (-6.367, 39.0865)
  line L61 (-6.367, 39.0865) -> (-4.5762, 39.0865)
  line L62 (-4.5762, 39.0865) -> (-4.5762, 38.4504)
  spline S42 degree 2 poles (-4.5762, 38.4504) (-4.1378, 38.8209) (-3.3042, 39.2408) (-2.7978, 39.2408) knots 0 0 0 1 2 2 2
  spline S43 degree 2 poles (-2.7978, 39.2408) (-1.921, 39.2408) (-0.9885, 38.1293) (-0.9885, 37.0796) knots 0 0 0 1 2 2 2
  line L63 (-0.9885, 37.0796) -> (-0.9885, 33.3375)
  spline S44 degree 2 poles (5.5632, 33.9982) (5.5632, 33.2016) (5.1001, 32.084) (4.7049, 31.7752) knots 0 0 0 1 2 2 2
  spline S45 degree 2 poles (4.7049, 31.7752) (4.3035, 31.4603) (3.192, 31.1762) (2.5127, 31.1762) knots 0 0 0 1 2 2 2
  spline S46 degree 2 poles (2.5127, 31.1762) (1.9384, 31.1762) (0.9072, 31.3244) (0.5305, 31.4232) knots 0 0 0 1 2 2 2
  line L64 (0.5305, 31.4232) -> (0.5305, 32.862)
  line L65 (0.5305, 32.862) -> (0.7405, 32.862)
  spline S47 degree 2 poles (0.7405, 32.862) (0.8702, 32.8126) (1.2345, 32.6891) (1.4197, 32.6397) knots 0 0 0 1 2 2 2
  spline S48 degree 2 poles (1.4197, 32.6397) (1.642, 32.5841) (2.0619, 32.51) (2.2781, 32.51) knots 0 0 0 1 2 2 2
  spline S49 degree 2 poles (2.2781, 32.51) (2.735, 32.51) (3.3402, 32.6953) (3.4946, 32.8682) knots 0 0 0 1 2 2 2
  spline S50 degree 2 poles (3.4946, 32.8682) (3.6489, 33.0473) (3.7724, 33.5289) (3.7724, 33.8994) knots 0 0 0 1 2 2 2
  line L66 (3.7724, 33.8994) -> (3.7724, 34.0044)
  spline S51 degree 2 poles (3.7724, 34.0044) (3.4699, 33.7389) (2.6795, 33.4178) (2.2596, 33.4178) knots 0 0 0 1 2 2 2
  spline S52 degree 2 poles (2.2596, 33.4178) (1.1419, 33.4178) (-0.0684, 34.8689) (-0.0684, 36.3571) knots 0 0 0 1 2 2 2
  spline S53 degree 2 poles (-0.0684, 36.3571) (-0.0684, 37.0302) (0.3021, 38.1046) (0.6355, 38.4813) knots 0 0 0 1 2 2 2
  spline S54 degree 2 poles (0.6355, 38.4813) (0.9566, 38.8456) (1.852, 39.2408) (2.3398, 39.2408) knots 0 0 0 1 2 2 2
  spline S55 degree 2 poles (2.3398, 39.2408) (2.7783, 39.2408) (3.476, 39.0185) (3.7601, 38.8333) knots 0 0 0 1 2 2 2
  line L67 (3.7601, 38.8333) -> (3.828, 39.0865)
  line L68 (3.828, 39.0865) -> (5.5632, 39.0865)
  line L69 (5.5632, 39.0865) -> (5.5632, 33.9982)
  line L70 (3.7724, 35.1468) -> (3.7724, 37.7527)
  spline S56 degree 2 poles (3.7724, 37.7527) (3.6428, 37.8144) (3.2537, 37.8947) (3.0561, 37.8947) knots 0 0 0 1 2 2 2
  spline S57 degree 2 poles (3.0561, 37.8947) (2.4139, 37.8947) (1.7655, 37.061) (1.7655, 36.3139) knots 0 0 0 1 2 2 2
  spline S58 degree 2 poles (1.7655, 36.3139) (1.7655, 35.9434) (1.8643, 35.4247) (1.994, 35.2271) knots 0 0 0 1 2 2 2
  spline S59 degree 2 poles (1.994, 35.2271) (2.1237, 35.0295) (2.5374, 34.8319) (2.8585, 34.8319) knots 0 0 0 1 2 2 2
  spline S60 degree 2 poles (2.8585, 34.8319) (3.0994, 34.8319) (3.5625, 34.9986) (3.7724, 35.1468) knots 0 0 0 1 2 2 2
  spline S61 degree 2 poles (8.6816, 33.1831) (8.0517, 33.1831) (6.9217, 33.461) (6.5512, 33.6463) knots 0 0 0 1 2 2 2
  line L71 (6.5512, 33.6463) -> (6.5512, 35.1591)
  line L72 (6.5512, 35.1591) -> (6.6994, 35.1591)
  spline S62 degree 2 poles (6.6994, 35.1591) (6.8291, 35.0603) (7.1564, 34.8257) (7.4466, 34.696) knots 0 0 0 1 2 2 2
  spline S63 degree 2 poles (7.4466, 34.696) (7.6998, 34.5787) (8.3234, 34.412) (8.6939, 34.412) knots 0 0 0 1 2 2 2
  spline S64 degree 2 poles (8.6939, 34.412) (9.0706, 34.412) (9.6511, 34.6466) (9.6511, 34.8998) knots 0 0 0 1 2 2 2
  spline S65 degree 2 poles (9.6511, 34.8998) (9.6511, 35.0974) (9.3855, 35.3073) (9.0027, 35.3938) knots 0 0 0 1 2 2 2
  spline S66 degree 2 poles (9.0027, 35.3938) (8.7989, 35.4494) (8.1752, 35.5667) (7.9344, 35.6408) knots 0 0 0 1 2 2 2
  spline S67 degree 2 poles (7.9344, 35.6408) (7.2552, 35.8507) (6.5759, 36.672) (6.5759, 37.3451) knots 0 0 0 1 2 2 2
  spline S68 degree 2 poles (6.5759, 37.3451) (6.5759, 37.728) (6.9279, 38.4072) (7.2737, 38.6727) knots 0 0 0 1 2 2 2
  spline S69 degree 2 poles (7.2737, 38.6727) (7.6133, 38.9321) (8.6198, 39.2408) (9.2559, 39.2408) knots 0 0 0 1 2 2 2
  spline S70 degree 2 poles (9.2559, 39.2408) (9.861, 39.2408) (10.8737, 39) (11.2195, 38.8333) knots 0 0 0 1 2 2 2
  line L73 (11.2195, 38.8333) -> (11.2195, 37.376)
  line L74 (11.2195, 37.376) -> (11.0775, 37.376)
  spline S71 degree 2 poles (11.0775, 37.376) (10.9849, 37.4501) (10.5835, 37.6909) (10.3983, 37.7774) knots 0 0 0 1 2 2 2
  spline S72 degree 2 poles (10.3983, 37.7774) (10.1698, 37.8762) (9.614, 38.012) (9.3238, 38.012) knots 0 0 0 1 2 2 2
  spline S73 degree 2 poles (9.3238, 38.012) (8.9348, 38.012) (8.3975, 37.7465) (8.3975, 37.5304) knots 0 0 0 1 2 2 2
  spline S74 degree 2 poles (8.3975, 37.5304) (8.3975, 37.3328) (8.6631, 37.1104) (9.1077, 36.9993) knots 0 0 0 1 2 2 2
  spline S75 degree 2 poles (9.1077, 36.9993) (9.3361, 36.9437) (9.9351, 36.8387) (10.213, 36.7461) knots 0 0 0 1 2 2 2
  spline S76 degree 2 poles (10.213, 36.7461) (10.8305, 36.5485) (11.4727, 35.7766) (11.4727, 35.1344) knots 0 0 0 1 2 2 2
  spline S77 degree 2 poles (11.4727, 35.1344) (11.4727, 34.7331) (11.096, 33.9982) (10.7441, 33.7512) knots 0 0 0 1 2 2 2
  spline S78 degree 2 poles (10.7441, 33.7512) (10.3797, 33.4795) (9.3794, 33.1831) (8.6816, 33.1831) knots 0 0 0 1 2 2 2
  point P0 (17.4625, -17.4625)
  constraints: 8 end point, 2 midpoint, 1 horizontal